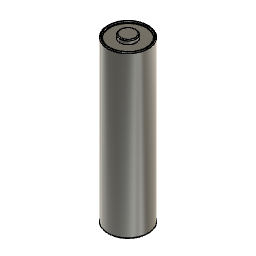
pilha 12v v1 (Autodesk Fusion 360 design; units mm, degrees)
Autodesk Fusion 360 part; units mm, degrees
sketch "Sketch1" plane through (0, 0, 0) normal (0, 0, 1) x (1, 0, 0)
  circle A0 centre (0, 0) radius 2.5
  dimension "d1" = 5
  constraint coincident A0.centre origin
  measures "d1" diameter of A0
extrude "Extrude1" add sketch "Sketch1" along normal blind 20
fillet "Fillet1" radius 0.1 1 edges at (-2.3308, -0.904, 0)
fillet "Fillet2" radius 0.1 1 edges at (-2.3308, -0.904, 20)
sketch "Sketch2" plane through (0, 0, 20) normal (0, 0, 1) x (-1, 0, 0)
  circle A0 centre (0, 0) radius 2.4
  circle A1 centre (0, 0) radius 2.25
  dimension "d8" = 4.5
  constraint coincident A0.centre A1.centre
  measures "d8" diameter of A1
extrude "Extrude2" cut sketch "Sketch2" against normal blind 0.2 contours A1
fillet "Fillet3" radius 0.1 1 edges at (2.0977, -0.8136, 20)
sketch "Sketch3" plane through (0, 0, 19.8) normal (0, 0, 1) x (-1, 0, 0)
  circle A0 centre (0, 0) radius 2.25
  circle A1 centre (0, 0) radius 1
  dimension "d13" = 2
  constraint coincident A0.centre A1.centre
  measures "d13" diameter of A1
extrude "Extrude3" add sketch "Sketch3" along normal blind 0.5 contours A1
fillet "Fillet4" radius 0.1 1 edges at (0.9323, 0.3616, 20.3)
